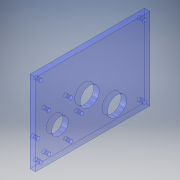
# Autodesk Inventor part: InsideMotorPlate
Saved by Autodesk Inventor 2019 (Build 230136000, 136)
## iProperties
Created: 2020-02-28
Part Number: InsideMotorPlate
Material: Aluminum 6061
Document SubType Name: Modeling
Designer: james
Density: 2.7 g/cm^3
Appearance: Clear - Blue
Mass: 134.969 g
Surface Area: 248.661 cm^2
Volume: 49.9883 cm^3
Author: james
Autodesk Inventor part; units mm, degrees
ref_plane "YZ Plane" through (0, 0, 0) normal (1, 0, 0) x (0, 1, 0)
ref_plane "XZ Plane" through (0, 0, 0) normal (0, 1, 0) x (-1, 0, 0)
ref_plane "XY Plane" through (0, 0, 0) normal (0, 0, 1) x (1, 0, 0)
sketch "Sketch1" plane through (0, 0, 0) normal (1, 0, 0) x (0, 1, 0)
  line L0 (46.7204, 78.4349) -> (-48.5296, 78.4349)
  line L1 (-48.5296, 78.4349) -> (-48.5296, -54.9151)
  line L2 (-48.5296, -54.9151) -> (46.7204, -54.9151)
  line L3 (46.7204, -54.9151) -> (46.7204, 78.4349)
  point P0 (0, 0)
  dimension "d0" = 133.35
  dimension "d1" = 95.25
  constraints: 8 end point, 2 parallel, 1 horizontal, 1 perpendicular
  measures "d0" distance of L2.end L0.start
  measures "d1" distance of L0.start L0.end
extrude "Extrusion1" add sketch "Sketch1" along normal blind 6.35
sketch "Sketch2" plane through (6.35, 0, 0) normal (1, 0, 0) x (0, 0, -1)
  line L0 (54.9151, 46.7204) -> (-78.4349, 46.7204) projected
  line L1 (-78.4349, 46.7204) -> (-78.4349, -48.5296) projected
  line L2 (-78.4349, -48.5296) -> (54.9151, -48.5296) projected
  line L3 (54.9151, -48.5296) -> (54.9151, 46.7204) projected
  point P0 (0, 0)
  point P1 (-72.0849, 40.3704)
  point P2 (48.5651, 40.3704)
  point P3 (48.5651, -42.1796)
  point P4 (-72.0849, -42.1796)
  dimension "d4" = 0
  dimension "d5" = 0
  dimension "d6" = 0
  dimension "d7" = 0
  dimension "d8" = 6.35
  dimension "d9" = 6.35
  dimension "d10" = 6.35
  dimension "d11" = 6.35
  measures "d4" horizontal distance of point (-72.085, -42.18) point (-72.085, 40.37)
  measures "d5" horizontal distance of point (48.565, 40.37) point (48.565, -42.18)
  measures "d6" vertical distance of point (-72.085, -42.18) point (48.565, -42.18)
  measures "d7" vertical distance of point (-72.085, 40.37) point (48.565, 40.37)
  measures "d8" distance from line of L0 point (-72.085, 40.37)
  measures "d9" distance from line of L1 point (-72.085, 40.37)
  measures "d10" distance from line of L2 point (-72.085, -42.18)
  measures "d11" distance from line of L3 point (48.565, -42.18)
hole "Hole1" at (6.35, 40.3704, 72.0849) at (6.35, 40.3704, -48.5651) at (6.35, -42.1796, -48.5651) at (6.35, -42.1796, 72.0849) direction (-1, 0, 0) diameter 4.318 end through all
sketch "Sketch3" plane through (6.35, 0, 0) normal (1, 0, 0) x (0, 0, -1)
  circle A0 centre (-49.8599, -16.7796) radius 9.652
  line L0 (-78.4349, -48.5296) -> (54.9151, -48.5296) projected
  line L1 (-78.4349, 46.7204) -> (-78.4349, -48.5296) projected
  point P0 (0, 0)
  dimension "d19" = 19.304
  dimension "d20" = 31.75
  dimension "d21" = 28.575
  constraints: 1 centre point
  measures "d19" diameter of A0
  measures "d20" distance from line of L0 A0.centre
  measures "d21" distance from line of L1 A0.centre
extrude "Extrusion2" cut sketch "Sketch3" against normal blind 61.9125
sketch "Sketch4" plane through (6.35, 0, 0) normal (1, 0, 0) x (0, 0, -1)
  circle A0 centre (-49.8599, -16.7796) radius 9.652 projected
  circle A1 centre (-49.8599, -16.7796) radius 9.652 projected
  circle A2 centre (-49.8599, -16.7796) radius 25.4
  line L0 (-49.8599, -16.7796) -> (-108.2264, -16.7796)
  line L1 (-49.8599, -16.7796) -> (-68.0839, 14.7853)
  line L2 (-49.8599, -16.7796) -> (-30.0658, 17.5048)
  line L3 (-49.8599, -16.7796) -> (-1.4138, -16.7796)
  line L4 (-49.8599, -16.7796) -> (-32.2617, -47.2605)
  line L5 (-49.8599, -16.7796) -> (-70.9793, -53.3594)
  point P0 (0, 0)
  point P1 (-75.2599, -16.7796)
  point P2 (-24.4599, -16.7796)
  point P3 (-62.5599, 5.2174)
  point P4 (-37.1599, 5.2174)
  point P5 (-37.1599, -38.7767)
  point P6 (-62.5599, -38.7767)
  dimension "d24" = 50.8
  dimension "d25" = 60
  dimension "d26" = 60
  dimension "d27" = 60
  dimension "d28" = 60
  constraints: 12 end point, 6 point on circle, 5 point on line, 2 horizontal, 1 centre point, 1 coincident
  measures "d24" diameter of A2
  measures "d25" angle of L0 L1
  measures "d26" angle of L1 L2
  measures "d27" angle of L4 L3
  measures "d28" angle of L5 L0
hole "Hole2" at (6.35, -16.7796, 75.2599) at (6.35, -16.7796, 24.4599) at (6.35, 5.2174, 62.5599) at (6.35, 5.2174, 37.1599) at (6.35, -38.7767, 37.1599) at (6.35, -38.7767, 62.5599) direction (-1, 0, 0) diameter 4.318 end through all
sketch "Sketch5" plane through (6.35, 0, 0) normal (1, 0, 0) x (0, 0, -1)
  circle A0 centre (-15.2888, -4.0796) radius 11.1125
  circle A1 centre (-49.8599, -16.7796) radius 9.652 projected
  circle A2 centre (-49.8599, -16.7796) radius 36.83
  point P0 (0, 0)
  dimension "d37" = 73.66
  dimension "d36" = 22.225
  dimension "d44" = 12.7
  constraints: 1 centre point, 1 coincident, 3 other
  measures "d36" diameter of A0
  measures "d44" vertical distance of A1.centre A0.centre
extrude "Extrusion3" cut sketch "Sketch5" against normal blind 66.675 contours A0 A2 | A2 A0 picked at (-12.0886, -2.4751) picked at (-18.8832, -5.4)
sketch "Sketch6" plane through (6.35, 0, 0) normal (1, 0, 0) x (0, 0, -1)
  circle A0 centre (-15.2888, -4.0796) radius 11.1125 projected
  circle A1 centre (-15.2888, -4.0796) radius 40.64
  circle A2 centre (16.4357, -29.4796) radius 11.1125
  line L0 (54.9151, 46.7204) -> (-78.4349, 46.7204) projected
  point P0 (0, 0)
  dimension "d43" = 81.28
  dimension "d40" = 22.225
  dimension "d76" = 76.2
  constraints: 1 centre point, 1 coincident, 3 other
  measures "d40" diameter of A2
  measures "d76" distance from line of A2.centre L0
extrude "Extrusion4" cut sketch "Sketch6" against normal blind 39.6875 contours A2 A1 | A1 A2 picked at (13.4558, -27.0938) picked at (19.1446, -31.8372)
body "Solid1"
